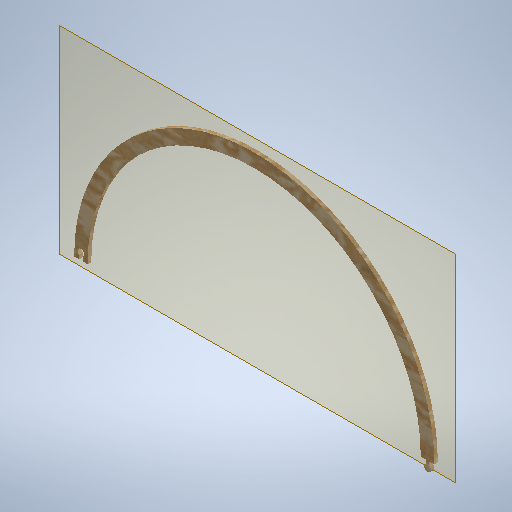
# Autodesk Inventor part: barrier
Saved by Autodesk Inventor 2025.2 (Build 292293000, 293)
## iProperties
Created: 2024-11-19
Part Number: barrier
Material: Generic
Document SubType Name: Modeling
Designer: jaros
Density: 1 g/cm^3
Appearance: Plywood - Weathered
Author: jaros
Autodesk Inventor part; units mm, degrees
ref_plane "YZ Plane" through (0, 0, 0) normal (1, 0, 0) x (0, 1, 0)
ref_plane "XZ Plane" through (0, 0, 0) normal (0, 1, 0) x (-1, 0, 0)
ref_plane "XY Plane" through (0, 0, 0) normal (0, 0, 1) x (1, 0, 0)
ref_plane "Work Plane1" through (0, 0, 0) normal (0, 0, 1) x (1, 0, 0)
sketch "Sketch1" plane through (0, 0, 0) normal (0, 0, 1) x (1, 0, 0)
  line L0 (250, -200) -> (400, -200) construction
  arc A0 (400, -200) -> (-400, -200) centre (0, -200) ccw construction
  line L1 (-400, -200) -> (-250, -200) construction
  arc A1 (250, -200) -> (-250, -200) centre (0, -200) ccw construction
  arc A2 (400, -200) -> (-400, -200) centre (0, -200) ccw
  arc A3 (370, -200) -> (-370, -200) centre (0, -200) ccw
  line L2 (400, -200) -> (370, -200) construction
  line L3 (385, -200) -> (385, -231.622) construction
  arc A4 (385, -222.5) -> (388.75, -208.5048) centre (385, -215) ccw
  line L4 (388.75, -208.5048) -> (388.75, -200)
  line L5 (400, -200) -> (388.75, -200)
  arc A5 (381.25, -208.5048) -> (385, -222.5) centre (385, -215) ccw
  line L6 (381.25, -208.5048) -> (381.25, -200)
  line L7 (370, -200) -> (381.25, -200)
  line L8 (-381.25, -191.4952) -> (-381.25, -200)
  arc A6 (-381.25, -191.4952) -> (-385, -177.5) centre (-385, -185) ccw
  line L9 (-370, -200) -> (-381.25, -200)
  arc A7 (-385, -177.5) -> (-388.75, -191.4952) centre (-385, -185) ccw
  line L10 (-388.75, -191.4952) -> (-388.75, -200)
  line L11 (-400, -200) -> (-388.75, -200)
  point P0 (0, 0)
  point P1 (-400, -200)
  point P2 (-370, -200)
  dimension "d0" = 30
  dimension "d1" = 7.5
  dimension "d2" = 7.5
  dimension "d3" = 15
  dimension "d6" = 180
  constraints: 20 end point, 12 point on circle, 6 centre point, 3 point on line, 2 perpendicular, 2 symmetric about line, 1 concentric, 1 midpoint, 1 vertical, 16 other
  measures "d0" radial gap between concentric circles of A0 A3
  measures "d1" radius of A4
  measures "d2" distance between parallel lines of L6 L4
  measures "d3" distance from line of A4.centre L0
extrude "Extrusion1" add sketch "Sketch1" along normal blind 8
body "Solid1"
